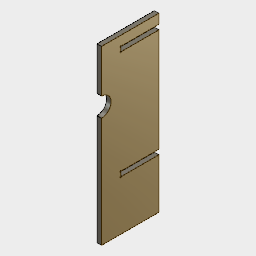
Support (Autodesk Fusion 360 design; units mm, degrees)
Autodesk Fusion 360 part; units mm, degrees
sketch "Sketch1" plane through (0, 0, 0) normal (1, 0, 0) x (0, 0, -1)
  line L0 (-15, 45) -> (15, 45)
  line L1 (15, 45) -> (15, -45)
  line L2 (15, -45) -> (-15, -45)
  line L3 (-15, -45) -> (-15, 45)
  line L4 (-15, 45) -> (15, -45) construction
  line L5 (15, 45) -> (-15, -45) construction
  dimension "d1" = 90
  dimension "d2" = 30
  constraint perpendicular L0 L1
  constraint parallel L0 L2
  constraint parallel L1 L3
  constraint horizontal L0
  constraint coincident L4
  constraint coincident L5
extrude "Extrude1" add sketch "Sketch1" along normal blind 2.4
sketch "Sketch3" plane through (2.4, 0, 0) normal (1, 0, 0) x (0, 0, -1)
  line L0 (-15, -45) -> (15, -45)
  line L1 (15, -45) -> (15, 45)
  line L2 (15, 45) -> (-15, 45)
  line L3 (-15, 45) -> (-15, -45)
  line L4 (15, 40) -> (-5, 40)
  line L5 (-5, 40) -> (-5, 37.5)
  line L6 (-5, 37.5) -> (15, 37.5)
  line L7 (15, 37.5) -> (15, 40)
  line L8 (15, -45) -> (15, 45)
  circle A0 centre (-5, 40) radius 0.375
  circle A1 centre (-5, 37.5) radius 0.375
  line L9 (15, -16.5) -> (-5, -16.5)
  circle A2 centre (-5, -16.5) radius 0.375
  line L10 (-5, -16.5) -> (-5, -19)
  circle A3 centre (-5, -19) radius 0.375
  line L11 (-5, -19) -> (15, -19)
  circle A4 centre (-15, 17.5) radius 5
  line L12 (-15, 45) -> (-15, -45)
  dimension "d18" = 2.5
  dimension "d19" = 20
  dimension "d20" = 5
  dimension "d21" = 0.75
  dimension "d22" = 0.75
  dimension "d25" = 0
  dimension "d26" = -56.5
  dimension "d28" = 10
  dimension "d29" = 20
  constraint horizontal L4
  constraint vertical L5
  constraint horizontal L6
  constraint vertical L7
  constraint coincident L1
  constraint coincident L3
  measures "d20" distance of L2
  measures "d21" diameter of A0
  measures "d22" diameter of A1
  measures "d28" diameter of A4
  measures "d29" distance of L6
extrude "Extrude3" cut sketch "Sketch3" against normal up to surface (2.4 mm away) contours L3 A4 L12 | L1 L8 L9 A2 L10 A3 L11 | L10 A3 L11 | L10 A3 L11 | L1 L4 L5 L6 L7 L8 A0 A1 | L9 A2 L10 | L9 A2 L10 | L5 L6 A1 | L5 L6 A1 | L4 L5 A0 | L4 L5 A0 picked at (-11.4083, 16.8879)
sketch "Sketch5" plane through (2.4, 0, 0) normal (1, 0, 0) x (0, 0, -1)
  arc A0 (-15, 12.5) -> (-15, 22.5) centre (-15, 17.5) ccw
  line L0 (-15, 12.5) -> (-15, -45)
  line L1 (-15, -45) -> (15, -45)
  line L2 (15, -45) -> (15, -19)
  line L3 (15, -19) -> (-4.625, -19)
  arc A1 (-5, -18.625) -> (-4.625, -19) centre (-5, -19) ccw
  line L4 (-5, -18.625) -> (-5, -16.875)
  arc A2 (-4.625, -16.5) -> (-5, -16.875) centre (-5, -16.5) ccw
  line L5 (-4.625, -16.5) -> (15, -16.5)
  line L6 (15, -16.5) -> (15, 37.5)
  line L7 (15, 37.5) -> (-4.625, 37.5)
  arc A3 (-5, 37.875) -> (-4.625, 37.5) centre (-5, 37.5) ccw
  line L8 (-5, 37.875) -> (-5, 39.625)
  arc A4 (-4.625, 40) -> (-5, 39.625) centre (-5, 40) ccw
  line L9 (-4.625, 40) -> (15, 40)
  line L10 (15, 40) -> (15, 45)
  line L11 (15, 45) -> (-15, 45)
  line L12 (-15, 45) -> (-15, 22.5)
